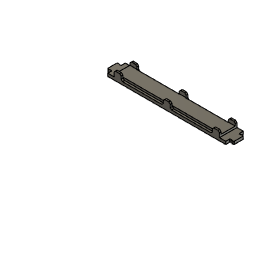
Sensor Bracket Bottom - Short Side (Autodesk Fusion 360 design; units mm, degrees)
Autodesk Fusion 360 part; units mm, degrees
sketch "Sketch1" plane through (0, 0, 0) normal (0, 1, 0) x (1, 0, 0)
  line L0 (125, 125) -> (-125, 125) construction
  line L1 (-125, 125) -> (-125, -125) construction
  line L2 (-125, -125) -> (125, -125) construction
  line L3 (125, -125) -> (125, 125) construction
  line L4 (125, 125) -> (-125, -125) construction
  line L5 (-125, 125) -> (125, -125) construction
  line L6 (75, 112.1152) -> (-75, 112.1152) construction
  line L7 (-75, 112.1152) -> (-75, 91.9152) construction
  line L8 (-75, 91.9152) -> (75, 91.9152) construction
  line L9 (75, 91.9152) -> (75, 112.1152) construction
  line L10 (75, 112.1152) -> (-75, 91.9152) construction
  line L11 (-75, 112.1152) -> (75, 91.9152) construction
  line L12 (137, 137) -> (92, 137)
  line L13 (92, 137) -> (137, 92)
  line L14 (137, 92) -> (137, 137)
  line L15 (125, 125) -> (137, 137) construction
  line L16 (128, 128) -> (109, 128) construction
  line L17 (109, 128) -> (128, 109) construction
  line L18 (128, 109) -> (128, 128) construction
  line L19 (92, 137) -> (84, 137)
  line L20 (84, 137) -> (84, 114)
  line L21 (84, 114) -> (104, 114)
  line L22 (104, 114) -> (114, 104)
  line L23 (114, 104) -> (114, 84)
  line L24 (114, 84) -> (137, 84)
  line L25 (137, 84) -> (137, 92)
  line L26 (84, 138) -> (-84, 138)
  line L27 (-84, 138) -> (-84, 113)
  line L28 (-84, 113) -> (84, 113)
  line L29 (84, 113) -> (84, 138)
  line L30 (84, 138) -> (-84, 113) construction
  line L31 (-84, 138) -> (84, 113) construction
  point P0 (0, 102.0152)
  point P1 (0, 125.5)
  dimension "d4" = 250
  dimension "d5" = 250
  dimension "d6" = 150
  dimension "d7" = 20.2
  dimension "d8" = 12
  dimension "d9" = 12
  dimension "d10" = 45
  dimension "d11" = 16
  dimension "d12" = 3
  dimension "d13" = 8
  dimension "d14" = 23
  dimension "d15" = 20
  dimension "d16" = 25
  dimension "d17" = 1
  constraint horizontal L0
  constraint perpendicular L0 L1
  constraint parallel L0 L2
  constraint parallel L1 L3
  constraint coincident L4 origin
  constraint coincident L5 origin
  constraint horizontal L6
  constraint perpendicular L6 L7
  constraint parallel L6 L8
  constraint parallel L7 L9
  constraint coincident L10 P0
  constraint coincident L11 P0
  constraint vertical origin P0
  constraint perpendicular L3 L12
  constraint perpendicular L4 L13
  constraint perpendicular L12 L14
  constraint parallel L4 L15
  constraint coincident L15 L16.start
  constraint parallel L12 L16
  constraint perpendicular L15 L17
  constraint perpendicular L16 L18
  constraint parallel L0 L19
  constraint perpendicular L0 L20
  constraint perpendicular L20 L21
  constraint parallel L13 L22
  constraint perpendicular L21 L23
  constraint perpendicular L23 L24
  constraint perpendicular L24 L25
  constraint equal L19 L25
  constraint equal L20 L24
  constraint horizontal L26
  constraint perpendicular L26 L27
  constraint parallel L26 L28
  constraint parallel L27 L29
  constraint coincident L30 P1
  constraint coincident L31 P1
  constraint coincident L20 L26.start
  constraint vertical origin P1
  measures "d4" distance of L1.end L2.end
  measures "d5" distance of L0.start L2.end
  measures "d6" distance of L6.start L6.end
  measures "d7" distance of L6 L8
  measures "d8" distance of L0 L12
  measures "d9" distance of L3 L14
  measures "d10" distance of L12.start L13.end
  measures "d11" horizontal distance of L0.start L16.end
  measures "d12" distance of L0 L16
  measures "d13" distance of L12.end L19.end
  measures "d14" distance of L19.end L20.end
  measures "d15" distance of L22.end L23.end
  measures "d16" distance of L26 L28
  measures "d17" distance of L19 L26
ref_plane "WorkPlane1" through (0, 7, 0) normal (0, 1, 0) x (0, 0, 1)
extrude "Extrude1" add sketch "Sketch1" along normal blind 4 contours L20 L26 L27 L28 L29
sketch "Sketch6" plane through (0, 4, 0) normal (0, 1, 0) x (-1, 0, 0)
  line L0 (-84, -113) -> (-84, -138)
  line L1 (-84, -138) -> (84, -138)
  line L2 (84, -138) -> (84, -113)
  line L3 (84, -113) -> (-84, -113)
  line L4 (-75, -135.575) -> (75, -135.575)
  line L5 (75, -135.575) -> (75, -115.425)
  line L6 (75, -115.425) -> (-75, -115.425)
  line L7 (-75, -115.425) -> (-75, -135.575)
  line L8 (-75, -135.575) -> (75, -115.425) construction
  line L9 (75, -135.575) -> (-75, -115.425) construction
  point P0 (0, -125.5)
  point P1 (0, -113)
  point P2 (84, -125.5)
  dimension "d36" = 150
  dimension "d37" = 20.15
  constraint horizontal L4
  constraint perpendicular L4 L5
  constraint parallel L4 L6
  constraint parallel L5 L7
  constraint coincident L8 P0
  constraint coincident L9 P0
  constraint midpoint L3 P1
  constraint vertical P0 P1
  constraint midpoint L2 P2
  constraint horizontal P0 P2
  measures "d36" distance of L4.start L4.end
  measures "d37" distance of L4.end L5.end
extrude "Extrude4" add sketch "Sketch6" along normal up to surface (3 mm away) contours L4 L5 L6 L7
sketch "Sketch7" plane through (0, 4, 0) normal (0, 1, 0) x (-1, 0, 0)
  line L0 (75, -135.575) -> (-75, -135.575)
  line L1 (-75, -135.575) -> (-75, -115.425)
  line L2 (-75, -115.425) -> (75, -115.425)
  line L3 (75, -115.425) -> (75, -135.575)
  line L4 (-84, -113) -> (-84, -138)
  line L5 (-84, -138) -> (84, -138)
  line L6 (84, -138) -> (84, -113)
  line L7 (84, -113) -> (-84, -113)
  line L8 (-5, -135.575) -> (5, -135.575)
  line L9 (5, -135.575) -> (5, -138)
  line L10 (5, -138) -> (-5, -138)
  line L11 (-5, -138) -> (-5, -135.575)
  line L12 (-5, -135.575) -> (5, -138) construction
  line L13 (5, -135.575) -> (-5, -138) construction
  line L14 (-5, -113) -> (5, -113)
  line L15 (5, -113) -> (5, -115.425)
  line L16 (5, -115.425) -> (-5, -115.425)
  line L17 (-5, -115.425) -> (-5, -113)
  line L18 (-5, -113) -> (5, -115.425) construction
  line L19 (5, -113) -> (-5, -115.425) construction
  line L20 (-75, -135.575) -> (-65, -135.575)
  line L21 (-65, -135.575) -> (-65, -138)
  line L22 (-65, -138) -> (-75, -138)
  line L23 (-75, -138) -> (-75, -135.575)
  line L24 (-75, -115.425) -> (-65, -115.425)
  line L25 (-65, -115.425) -> (-65, -113)
  line L26 (-65, -113) -> (-75, -113)
  line L27 (-75, -113) -> (-75, -115.425)
  line L28 (75, -135.575) -> (65, -135.575)
  line L29 (65, -135.575) -> (65, -138)
  line L30 (65, -138) -> (75, -138)
  line L31 (75, -138) -> (75, -135.575)
  line L32 (75, -115.425) -> (65, -115.425)
  line L33 (65, -115.425) -> (65, -113)
  line L34 (65, -113) -> (75, -113)
  line L35 (75, -113) -> (75, -115.425)
  point P0 (0, -136.7875)
  point P1 (0, -114.2125)
  dimension "d42" = 10
  constraint horizontal L8
  constraint perpendicular L8 L9
  constraint parallel L8 L10
  constraint parallel L9 L11
  constraint coincident L12 P0
  constraint coincident L13 P0
  constraint coincident L0 L8.start
  constraint horizontal L14
  constraint perpendicular L14 L15
  constraint parallel L14 L16
  constraint parallel L15 L17
  constraint coincident L18 P1
  constraint coincident L19 P1
  constraint coincident L7 L14.start
  constraint vertical P0 P1
  constraint vertical origin P1
  constraint equal L10 L16
  constraint coincident L2 L16.end
  constraint coincident L5 L10.end
  constraint horizontal L20
  constraint vertical L21
  constraint horizontal L22
  constraint vertical L23
  constraint coincident L5 L21.end
  constraint coincident L0.end L1.start
  constraint horizontal L24
  constraint vertical L25
  constraint horizontal L26
  constraint vertical L27
  constraint coincident L7 L25.end
  constraint coincident L1.end L2.start
  constraint horizontal L28
  constraint vertical L29
  constraint horizontal L30
  constraint vertical L31
  constraint coincident L5 L29.end
  constraint coincident L0.start L3.end
  constraint horizontal L32
  constraint vertical L33
  constraint horizontal L34
  constraint vertical L35
  constraint coincident L7 L33.end
  constraint coincident L2.end L3.start
  constraint equal L30 L34
  constraint equal L22 L30
  constraint equal L22 L26
  constraint equal L10 L22
  measures "d42" distance of L15.end L16.end
extrude "Extrude5" add sketch "Sketch7" along normal blind 8 contours L0 L5 L28 L29 L30 L31 | L2 L7 L32 L33 L34 L35 | L0 L5 L8 L9 L10 L11 | L2 L7 L14 L15 L16 L17 | L0 L5 L20 L21 L22 L23 | L2 L7 L24 L25 L26 L27
chamfer "Chamfer1" distance 2 angle 45 12 edges at (-5, 12, -136.7875) (5, 12, -136.7875) (-5, 12, -114.2125) (5, 12, -114.2125) (-75, 12, -136.7875) (-65, 12, -136.7875) (-75, 12, -114.2125) (-65, 12, -114.2125) (65, 12, -136.7875) (75, 12, -136.7875) (65, 12, -114.2125) (75, 12, -114.2125)
sketch "Sketch9" plane through (0, 0, 0) normal (0, -1, 0) x (1, 0, 0)
  line L0 (84, -138) -> (84, -113)
  line L1 (84, -113) -> (-84, -113)
  line L2 (-84, -113) -> (-84, -138)
  line L3 (-84, -138) -> (84, -138)
  line L4 (84, -119.5) -> (90, -118)
  line L5 (90, -118) -> (90, -133)
  line L6 (90, -133) -> (84, -131.5)
  line L7 (90, -118) -> (84, -131.5) construction
  line L8 (90, -133) -> (84, -119.5) construction
  line L9 (90, -125.5) -> (84, -125.5) construction
  line L10 (84.0049, -119.5194) -> (89.98, -118.0256)
  line L11 (89.98, -118.0256) -> (89.98, -132.9744)
  line L12 (89.98, -132.9744) -> (84.0049, -131.4806)
  line L13 (84.0049, -131.4806) -> (84, -131.4794)
  line L14 (84.0049, -119.5194) -> (84, -119.5206)
  point P0 (90, -125.5)
  dimension "d51" = 12
  dimension "d52" = 15
  dimension "d53" = 6
  dimension "d56" = 0.02
  constraint coincident L0 L4.start
  constraint parallel L0 L5
  constraint coincident L0 L6.end
  constraint equal L7 L8
  constraint midpoint L5 P0
  constraint coincident P0 L9.start
  constraint midpoint L0 L9.end
  constraint horizontal L9
  constraint coincident L0 L13.end
  constraint parallel L12 L13
  constraint coincident L0 L14.end
  constraint parallel L10 L14
  measures "d51" distance of L4.start L6.end
  measures "d52" distance of L4.end L5.end
  measures "d53" distance of L0 L4.end
extrude "Extrude7" add sketch "Sketch9" against normal blind 4 contours L0 L10 L11 L12 L13 L14
mirror "Mirror2" about plane through (0, 0, 0) normal (1, 0, 0) of "Extrude7"
fillet "Fillet2" radius 1 8 edges at (-84, 2, -119.5206) (-89.98, 2, -118.0256) (-84, 2, -131.4794) (-89.98, 2, -132.9744) (84, 2, -119.5206) (89.98, 2, -118.0256) (89.98, 2, -132.9744) (84, 2, -131.4794)
sketch "Sketch11" plane through (0, 7, 0) normal (0, 1, 0) x (-1, 0, 0)
  line L0 (-65, -115.425) -> (-75, -115.425)
  line L1 (-75, -115.425) -> (-75, -135.575)
  line L2 (-75, -135.575) -> (-65, -135.575)
  line L3 (-65, -135.575) -> (-5, -135.575)
  line L4 (-5, -135.575) -> (5, -135.575)
  line L5 (5, -135.575) -> (65, -135.575)
  line L6 (65, -135.575) -> (75, -135.575)
  line L7 (75, -135.575) -> (75, -115.425)
  line L8 (75, -115.425) -> (65, -115.425)
  line L9 (65, -115.425) -> (5, -115.425)
  line L10 (5, -115.425) -> (-5, -115.425)
  line L11 (-5, -115.425) -> (-65, -115.425)
  line L12 (65, -135.575) -> (5, -135.575)
  line L13 (5, -135.575) -> (5, -135.075)
  line L14 (5, -135.075) -> (65, -135.075)
  line L15 (65, -135.075) -> (65, -135.575)
  line L16 (65, -115.425) -> (5, -115.425)
  line L17 (5, -115.425) -> (5, -115.925)
  line L18 (5, -115.925) -> (65, -115.925)
  line L19 (65, -115.925) -> (65, -115.425)
  line L20 (-65, -135.575) -> (-5, -135.575)
  line L21 (-5, -135.575) -> (-5, -135.075)
  line L22 (-5, -135.075) -> (-65, -135.075)
  line L23 (-65, -135.075) -> (-65, -135.575)
  line L24 (-65, -115.425) -> (-5, -115.425)
  line L25 (-5, -115.425) -> (-5, -115.925)
  line L26 (-5, -115.925) -> (-65, -115.925)
  line L27 (-65, -115.925) -> (-65, -115.425)
  dimension "d63" = 0.5
  constraint horizontal L12
  constraint vertical L13
  constraint horizontal L14
  constraint vertical L15
  constraint coincident L5.end L6.start
  constraint horizontal L16
  constraint vertical L17
  constraint horizontal L18
  constraint vertical L19
  constraint coincident L8.end L9.start
  constraint horizontal L20
  constraint vertical L21
  constraint horizontal L22
  constraint vertical L23
  constraint coincident L2.end L3.start
  constraint horizontal L24
  constraint vertical L25
  constraint horizontal L26
  constraint vertical L27
  constraint coincident L0.start L11.end
  constraint coincident L10.end L11.start
  constraint coincident L3.end L4.start
  constraint coincident L4.end L5.start
  constraint coincident L9.end L10.start
  constraint equal L13 L21
  constraint equal L21 L25
  constraint equal L17 L25
  measures "d63" distance of L10.end L25.end
extrude "Extrude8" cut sketch "Sketch11" against normal blind 3 contours L11 L24 L25 L26 L27 | L9 L16 L17 L18 L19 | L3 L20 L21 L22 L23 | L5 L12 L13 L14 L15
chamfer "Chamfer2" distance 2 angle 45 8 edges at (5, 4, -114.4625) (-5, 4, -114.4625) (-5, 4, -136.5375) (65, 4, -136.5375) (65, 4, -114.4625) (5, 4, -136.5375) (-65, 4, -114.4625) (-65, 4, -136.5375)
equation "sensor_ref = 7 mm"
